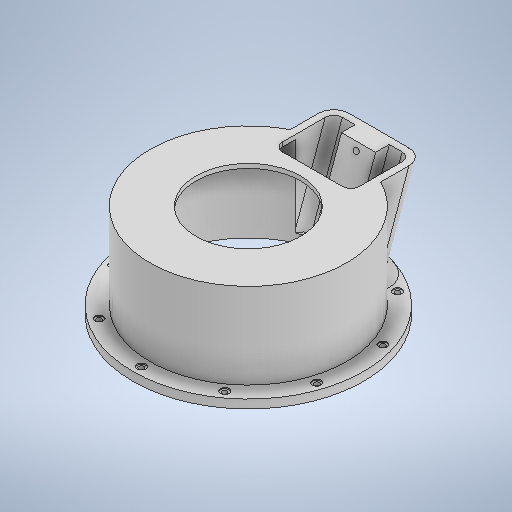
# Autodesk Inventor part: Vibrometer Housing
Saved by Autodesk Inventor 2026.2 (Build 302298000, 298)
## iProperties
Created: 2026-03-24
Part Number: Vibrometer Housing
Material: Generic
Document SubType Name: Modeling
Designer: mumin
Density: 1 g/cm^3
Appearance: Default
Author: mumin
Autodesk Inventor part; units mm, degrees
ref_plane "YZ Plane" through (0, 0, 0) normal (1, 0, 0) x (0, 1, 0)
ref_plane "XZ Plane" through (0, 0, 0) normal (0, 1, 0) x (-1, 0, 0)
ref_plane "XY Plane" through (0, 0, 0) normal (0, 0, 1) x (1, 0, 0)
sketch "Sketch1" plane through (0, 0, 0) normal (1, 0, 0) x (0, 1, 0)
  line L0 (0, 0) -> (120, 0)
  line L1 (110, -61.25) -> (105, -61.25)
  line L2 (105, -61.25) -> (105, -110)
  line L3 (105, -110) -> (0, -110)
  line L4 (0, -110) -> (0, -135)
  line L5 (0, -135) -> (10, -135)
  line L6 (10, -135) -> (10, -115)
  line L7 (10, -115) -> (110, -115)
  line L8 (110, -115) -> (110, -61.25)
  line L9 (0, -114) -> (2, -114)
  line L10 (2, -114) -> (2, -117)
  line L11 (2, -117) -> (0, -117)
  line L12 (0, -117) -> (0, -114)
  point P0 (2, -115)
  point P1 (1, -114)
  dimension "d1" = 270
  dimension "d2" = 220
  dimension "d3" = 230
  dimension "d4" = 122.5
  dimension "d5" = 10
  dimension "d6" = 5
  dimension "d7" = 110
  dimension "d21" = 228
  dimension "d22" = 3
  dimension "d24" = 2
  constraints: 26 end point, 8 perpendicular, 3 horizontal, 2 parallel, 2 point on line
  measures "d1" diameter of L5 L0
  measures "d2" diameter of L3 L0
  measures "d3" diameter of L7 L0
  measures "d4" diameter of L1 L0
  measures "d5" distance between parallel lines of L4 L6
  measures "d6" distance between parallel lines of L2 L8
  measures "d7" distance between parallel lines of L4 L8
  measures "d21" diameter of L9 L0
  measures "d22" distance of L9.end L10.end
  measures "d24" distance from line of L4 L10.end
revolve "Base Cylinder" add sketch "Sketch1" angle 360 about axis through (0, 0, 0) along (0, 1, 0)
sketch "Sketch2" plane through (0, 10, 0) normal (0, 1, 0) x (1, 0, 0)
  point P0 (0, 0)
  point P1 (0, 125)
  point P2 (-73.4732, 101.1271)
  point P3 (-118.8821, 38.6271)
  point P4 (-118.8821, -38.6271)
  point P5 (-73.4732, -101.1271)
  point P6 (0, -125)
  point P7 (73.4732, -101.1271)
  point P8 (118.8821, -38.6271)
  point P9 (118.8821, 38.6271)
  point P10 (73.4732, 101.1271)
  dimension "d9" = 125
  dimension "d12" = 360
  constraints: 11 other
  measures "d9" distance of point (0, 0) point (0, 125)
hole "M5 Mounting Holes" at (0, 10, -125) at (-73.4732, 10, -101.1271) at (-118.8821, 10, -38.6271) at (-118.8821, 10, 38.6271) at (-73.4732, 10, 101.1271) at (0, 10, 125) at (73.4732, 10, 101.1271) at (118.8821, 10, 38.6271) at (118.8821, 10, -38.6271) at (73.4732, 10, -101.1271) direction (0, -1, 0) diameter 5.9 end through all counterbore diameter 10.2 counterbore depth 1.2
sketch "Sketch3" plane through (0, 110, 0) normal (0, 1, 0) x (1, 0, 0)
  line L0 (0, 143.2495) -> (0, 0)
  circle A0 centre (0, 0) radius 61.25 projected
  circle A1 centre (0, 0) radius 115 projected
  line L1 (-45, 105.8301) -> (-45, 85)
  line L2 (0, 75) -> (-35, 75)
  arc A2 (-45, 85) -> (-35, 75) centre (-35, 85) ccw
  line L3 (45, 105.8301) -> (45, 85)
  line L4 (0, 75) -> (35, 75)
  arc A3 (35, 75) -> (45, 85) centre (35, 85) ccw
  point P0 (45, 105.8301)
  dimension "d25" = 10
  dimension "d26" = 90
  dimension "d27" = 75
  constraints: 10 end point, 4 point on circle, 4 symmetric about line, 2 centre point, 2 tangent, 2 vertical, 1 perpendicular, 1 point on line, 3 other
  measures "d25" radius of A2
  measures "d26" diameter of L1 L0
  measures "d27" distance from line of L0.end L2
extrude "Access Cutout" cut sketch "Sketch3" against normal up to surface (100 mm away) contours A1 L3 A3 L4 L0 | L0 L2 A2 L1 A1
sketch "Sketch4" plane through (0, 110, 0) normal (0, 1, 0) x (1, 0, 0)
  line L0 (45, 105.8301) -> (45, 85) projected
  arc A0 (35, 75) -> (45, 85) centre (35, 85) ccw projected
  line L1 (35, 75) -> (-35, 75) projected
  arc A1 (-45, 85) -> (-35, 75) centre (-35, 85) ccw projected
  line L2 (-45, 85) -> (-45, 105.8301) projected
  arc A2 (-45, 105.8301) -> (45, 105.8301) centre (0, 0) ccw projected
  circle A3 centre (0, 0) radius 61.25 projected
  line L3 (0, 0) -> (0, 180)
  line L4 (-45, 105.8301) -> (-45, 135)
  line L5 (-35, 145) -> (0, 145)
  arc A4 (-35, 145) -> (-45, 135) centre (-35, 135) ccw
  line L6 (0, 153) -> (-35, 153)
  arc A5 (-35, 153) -> (-53, 135) centre (-35, 135) ccw
  line L7 (-53, 135) -> (-53, 102.0588)
  line L8 (45, 105.8301) -> (45, 135)
  line L9 (35, 145) -> (0, 145)
  arc A6 (45, 135) -> (35, 145) centre (35, 135) ccw
  line L10 (0, 153) -> (35, 153)
  arc A7 (53, 135) -> (35, 153) centre (35, 135) ccw
  line L11 (53, 135) -> (53, 102.0588)
  dimension "d31" = 10
  dimension "d32" = 8
  dimension "d33" = 145
  constraints: 18 end point, 9 point on circle, 6 symmetric about line, 4 centre point, 2 tangent, 2 vertical, 1 parallel, 1 perpendicular, 1 point on line, 3 other
  measures "d31" radius of A4
  measures "d32" distance between parallel lines of L5 L6
  measures "d33" distance from line of point (0, 0) L5
sketch "Sketch5" plane through (0, 0, 0) normal (1, 0, 0) x (0, 1, 0)
  line L0 (10, -96.0271) -> (10, -106.2271) projected
  line L1 (10, -33.5271) -> (10, -43.7271) projected
  line L2 (10, 43.7271) -> (10, 33.5271) projected
  line L3 (10, 106.2271) -> (10, 96.0271) projected
  line L4 (10, 130.1) -> (10, 119.9) projected
  line L5 (10, 106.2271) -> (10, 96.0271) projected
  line L6 (10, 43.7271) -> (10, 33.5271) projected
  line L7 (10, -33.5271) -> (10, -43.7271) projected
  line L8 (10, -96.0271) -> (10, -106.2271) projected
  line L9 (10, -119.9) -> (10, -130.1) projected
  line L10 (10, -105.8301) -> (10, -105.8301) projected
  line L11 (10, -100.3743) -> (10, -105.8301) projected
  line L12 (10, -100.3743) -> (10, -100.3743) projected
  line L13 (10, -105.8301) -> (10, -100.3743) projected
  line L14 (10, -135) -> (10, 135) projected
  line L15 (110, -153) -> (10, -116.603)
  point P0 (0, 0)
  dimension "d34" = 70
  constraints: 2 end point, 1 point on line
  measures "d34" angle of L14 L15
sweep "Angle Bracket" add profiles "Sketch4" path "Sketch5" keep normal constant yes path curves L15 contours L8 A6 L9 L3 L10 A7 L11 A2 | L7 A5 L6 L3 L5 A4 L4 A2
sketch "Sketch6" plane through (0, 105, 0) normal (0, -1, 0) x (1, 0, 0)
  line L0 (45, -85) -> (45, -100.3743) projected
  arc A0 (45, -100.3743) -> (-45, -100.3743) centre (0, 0) ccw projected
  line L1 (-45, -100.3743) -> (-45, -85) projected
  arc A1 (-35, -75) -> (-45, -85) centre (-35, -85) ccw projected
  line L2 (-35, -75) -> (35, -75) projected
  arc A2 (45, -85) -> (35, -75) centre (35, -85) ccw projected
  circle A3 centre (0, 0) radius 61.25 projected
  arc A4 (-45, -100.3743) -> (45, -100.3743) centre (0, 0) ccw
  constraints: 2 point on circle, 1 centre point, 1 coincident
extrude "Remove Material (Sweep)" cut sketch "Sketch6" along normal up to surface (105 mm away)
sketch "Sketch7" plane through (0, 0, 0) normal (0, -1, 0) x (1, 0, 0)
  circle A0 centre (0, -125) radius 5.1 projected
  point P0 (0, 0)
extrude "Fill Extra Hole" add sketch "Sketch7" against normal up to surface (10 mm away)
sketch "Sketch8" plane through (-35, 110, -145) normal (0, 0.3420201, 0.9396926) x (1, 0, 0)
  line L0 (35, -152.9591) -> (35, 19.858)
  line L1 (15, -90) -> (55, -90)
  line L2 (55, -90) -> (55, 0)
  line L3 (55, 0) -> (15, 0)
  line L4 (15, 0) -> (15, -90)
  line L5 (15, -90) -> (55, 0) construction
  line L6 (55, -90) -> (15, 0) construction
  line L7 (0, 0) -> (70, 0) projected
  point P0 (35, -45)
  point P1 (35, 0)
  dimension "d41" = 90
  dimension "d42" = 40
  constraints: 14 end point, 4 midpoint, 2 parallel, 1 horizontal, 1 perpendicular, 1 point on line, 1 vertical
  measures "d41" distance between parallel lines of L7 L1
  measures "d42" distance between parallel lines of L2 L4
extrude "Riser Mount" add sketch "Sketch8" along normal blind 15
sketch "Sketch9" plane through (35, 110, -153) normal (0, -0.3420201, -0.9396926) x (-1, 0, 0)
  line L0 (35, -155.6953) -> (35, 12.0569)
  line L1 (0, 0) -> (70, 0) projected
  point P0 (35, -59)
  point P1 (35, -16)
  dimension "d47" = 59
  dimension "d57" = 43
  constraints: 2 end point, 2 point on line, 1 vertical
  measures "d47" distance from line of L1 point (35, -59)
  measures "d57" distance of point (35, -59) point (35, -16)
hole "M6 & 1/4-20 Mount Holes" at (0, 54.5581, -132.8208) direction (0, 0.3420201, 0.9396926) diameter 5.5 depth 22.5175 counterbore diameter 10.1 counterbore depth 1.2
sketch "Sketch10" plane through (20, 25.4277, -114.2182) normal (1, 0, 0) x (0, -0.3420201, -0.9396926)
  line L0 (-40.3515, 75.3132) -> (-9.3969, 86.5798) projected
  line L1 (0, 90) -> (0, 0) projected
  line L2 (0, 90) -> (-15, 90) projected
  line L3 (-15, 0) -> (-15, 90) projected
  line L4 (0, 0) -> (-15, 0) projected
  line L5 (0, 90) -> (-15, 90)
  line L6 (-15, 84.5404) -> (0, 90)
  point P0 (-98.6332, -62.9591)
  point P1 (-9.3969, 86.5798)
  constraints: 4 end point, 2 collinear, 2 point on line
extrude "Remove Material (Riser Mount)" cut sketch "Sketch10" against normal up to surface (40 mm away) contours L3 L2 L6 L0
hole "Hole3" at (0, 94.9649, -147.5277) direction (0, 0.3420201, 0.9396926) diameter 6.7 depth 22.5175 counterbore diameter 12 counterbore depth 1.2
chamfer "Chamfer1" distance 10 angle 45 1 edges at (0, 30.558, -100.1228)
chamfer "Chamfer2" distance 5 angle 45 1 edges at (0, 25.4277, -114.2182)
chamfer "Chamfer3" distance 12 angle 45 3 edges at (46.3648, 10, -112.5615) (0, 10, -116.603) (-46.3648, 10, -112.5615)
body "Solid1"
